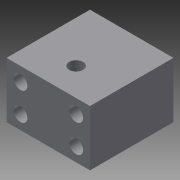
# Autodesk Inventor part: rod guide
Saved by Autodesk Inventor 2014 SP1 (Build 180222100, 222)
## iProperties
Created: 2014-02-07
Part Number: rod guide
Material: Generic
Document SubType Name: Modeling
Designer: Owner
Density: 1 g/cm^3
Appearance: Default
Author: Owner
Autodesk Inventor part; units mm, degrees
ref_plane "YZ Plane" through (0, 0, 0) normal (1, 0, 0) x (0, 1, 0)
ref_plane "XZ Plane" through (0, 0, 0) normal (0, 1, 0) x (-1, 0, 0)
ref_plane "XY Plane" through (0, 0, 0) normal (0, 0, 1) x (1, 0, 0)
sketch "Sketch1" plane through (0, 0, 0) normal (0, 0, 1) x (1, 0, 0)
  line L0 (-19.05, -12.7) -> (19.05, -12.7)
  line L1 (19.05, -12.7) -> (19.05, 12.7)
  line L2 (19.05, 12.7) -> (-19.05, 12.7)
  line L3 (-19.05, 12.7) -> (-19.05, -12.7)
  line L4 (-19.05, -12.7) -> (19.05, 12.7) construction
  line L5 (19.05, -12.7) -> (-19.05, 12.7) construction
  point P0 (0, 0)
  dimension "d0" = 38.1
  dimension "d1" = 25.4
  constraints: 12 end point, 2 midpoint, 2 parallel, 1 horizontal, 1 perpendicular
  measures "d0" distance of L2.end L1.end
  measures "d1" distance of L1.end L0.end
extrude "Extrusion1" add sketch "Sketch1" along normal blind 38.1
sketch "Sketch2" plane through (0, 0, 38.1) normal (0, 0, 1) x (1, 0, 0)
  line L0 (12.7, -6.35) -> (-12.7, -6.35)
  line L1 (-12.7, -6.35) -> (-12.7, 6.35)
  line L2 (-12.7, 6.35) -> (12.7, 6.35)
  line L3 (12.7, 6.35) -> (12.7, -6.35)
  line L4 (12.7, -6.35) -> (-12.7, 6.35) construction
  line L5 (-12.7, -6.35) -> (12.7, 6.35) construction
  point P0 (0, 0)
  point P1 (0, 0)
  dimension "d4" = 25.4
  dimension "d5" = 12.7
  constraints: 12 end point, 2 midpoint, 2 parallel, 1 coincident, 1 horizontal, 1 perpendicular
  measures "d4" distance of L1.end L2.end
  measures "d5" distance of L0.end L1.end
hole "Hole1" at (12.7, 6.35, 38.1) at (-12.7, 6.35, 38.1) at (-12.7, -6.35, 38.1) at (12.7, -6.35, 38.1) direction (0, 0, -1) diameter 6.35 end through all
sketch "Sketch3" plane through (-19.05, 12.7, 0) normal (0, 1, 0) x (1, 0, 0)
  line L0 (38.1, 0) -> (38.1, -38.1) projected
  line L1 (19.05, 0) -> (19.05, -25.4) construction
  dimension "d13" = 25.4
  constraints: 2 end point, 1 parallel
  measures "d13" distance of L1.start L1.end
hole "Hole2" at (0, 12.7, 25.4) direction (0, -1, 0) diameter 6.35 end through all
body "Solid1"
